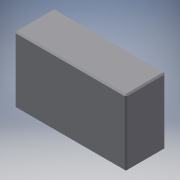
# Autodesk Inventor part: kloc
Saved by Autodesk Inventor 2018.3 (Build 223284000, 284)
## iProperties
Created: 2020-04-19
Part Number: kloc
Material: Ogólny
Document SubType Name: Modeling
Designer: Wojciech
Density: 1 g/cm^3
Appearance: Domyślna
Author: Wojciech
Autodesk Inventor part; units mm, degrees
ref_plane "YZ Plane" through (0, 0, 0) normal (1, 0, 0) x (0, 1, 0)
ref_plane "XZ Plane" through (0, 0, 0) normal (0, 1, 0) x (-1, 0, 0)
ref_plane "XY Plane" through (0, 0, 0) normal (0, 0, 1) x (1, 0, 0)
sketch "Szkic1" plane through (0, 0, 0) normal (0, 1, 0) x (-1, 0, 0)
  line L0 (-21, -12.5) -> (21, -12.5)
  line L1 (21, -12.5) -> (21, 12.5)
  line L2 (21, 12.5) -> (-21, 12.5)
  line L3 (-21, 12.5) -> (-21, -12.5)
  line L4 (-21, -12.5) -> (21, 12.5) construction
  line L5 (21, -12.5) -> (-21, 12.5) construction
  point P0 (0, 0)
  dimension "d2" = 42
  dimension "d3" = 25
  constraints: 12 end point, 2 midpoint, 2 parallel, 1 horizontal, 1 perpendicular
  measures "d2" distance of L1.end L2.end
  measures "d3" distance of L0.end L1.end
extrude "Wyciągnięcie proste1" add sketch "Szkic1" along normal blind 15
chamfer "Faza1" distance 0.5 angle 45 12 edges at (0, 15, -12.5) (0, 0, -12.5) (-21, 7.5, -12.5) (-21, 15, 0) (-21, 0, 0) (-21, 7.5, 12.5) (0, 15, 12.5) (0, 0, 12.5) (21, 7.5, 12.5) (21, 15, 0) (21, 7.5, -12.5) (21, 0, 0)
